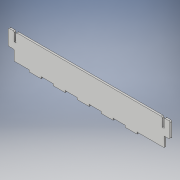
# Autodesk Inventor part: back_v2
Saved by Autodesk Inventor 2017.2 (Build 212233000, 233)
## iProperties
Created: 2017-06-09
Part Number: back_v2
Material: Generic
Document SubType Name: Modeling
Designer: SandeepSH
Density: 1 g/cm^3
Appearance: Default
Author: SandeepSH
Autodesk Inventor part; units mm, degrees
ref_plane "YZ Plane" through (0, 0, 0) normal (1, 0, 0) x (0, 1, 0)
ref_plane "XZ Plane" through (0, 0, 0) normal (0, 1, 0) x (-1, 0, 0)
ref_plane "XY Plane" through (0, 0, 0) normal (0, 0, 1) x (1, 0, 0)
sketch "Sketch1" plane through (0, 0, 0) normal (0, 0, 1) x (1, 0, 0)
  line L0 (0, 0) -> (250, 0)
  line L1 (250, 0) -> (250, 46)
  line L2 (250, 46) -> (0, 46)
  line L3 (0, 46) -> (0, 0)
  dimension "d0" = 250
  dimension "d1" = 46
  constraints: 8 end point, 2 parallel, 1 horizontal, 1 perpendicular
  measures "d0" distance of L2.end L1.end
  measures "d1" distance of L1.end L0.end
extrude "Extrusion1" add sketch "Sketch1" along normal blind 3
sketch "Sketch2" plane through (0, 0, 3) normal (0, 0, 1) x (1, 0, 0)
  line L0 (0, 0) -> (25, 0)
  line L1 (25, 0) -> (25, 3)
  line L2 (25, 3) -> (0, 3)
  line L3 (0, 3) -> (0, 0)
  line L4 (0, 0) -> (250, 0) projected
  line L5 (45, 0) -> (65, 0)
  line L6 (65, 0) -> (65, 3)
  line L7 (65, 3) -> (45, 3)
  line L8 (45, 3) -> (45, 0)
  line L9 (85, 0) -> (105, 0)
  line L10 (105, 0) -> (105, 3)
  line L11 (105, 3) -> (85, 3)
  line L12 (85, 3) -> (85, 0)
  line L13 (125, 0) -> (145, 0)
  line L14 (145, 0) -> (145, 3)
  line L15 (145, 3) -> (125, 3)
  line L16 (125, 3) -> (125, 0)
  line L17 (165, 0) -> (185, 0)
  line L18 (185, 0) -> (185, 3)
  line L19 (185, 3) -> (165, 3)
  line L20 (165, 3) -> (165, 0)
  line L21 (250, 0) -> (205, 0)
  line L22 (205, 0) -> (205, 3)
  line L23 (205, 3) -> (250, 3)
  line L24 (250, 3) -> (250, 0)
  dimension "d4" = 25
  dimension "d5" = 3
  dimension "d6" = 20
  dimension "d7" = 3
  dimension "d8" = 20
  dimension "d9" = 20
  dimension "d10" = 3
  dimension "d11" = 20
  dimension "d12" = 20
  dimension "d13" = 3
  dimension "d14" = 20
  dimension "d15" = 20
  dimension "d16" = 3
  dimension "d17" = 20
  dimension "d18" = 3
  dimension "d19" = 20
  constraints: 48 end point, 12 parallel, 6 horizontal, 6 perpendicular, 3 point on line, 1 midpoint
  measures "d4" distance of L2.end L1.end
  measures "d5" distance of L1.end L0.end
  measures "d6" distance of L7.end L6.end
  measures "d7" distance of L6.end L5.end
  measures "d8" distance between parallel lines of L8 L1
  measures "d9" distance of L11.end L10.end
  measures "d10" distance of L10.end L9.end
  measures "d11" distance from line of L11.end L6
  measures "d12" distance of L15.end L14.end
  measures "d13" distance of L14.end L13.end
  measures "d14" distance between parallel lines of L16 L10
  measures "d15" distance of L19.end L18.end
  measures "d16" distance of L18.end L17.end
  measures "d17" distance between parallel lines of L20 L14
  measures "d18" distance of L21.end L22.end
  measures "d19" distance between parallel lines of L22 L18
extrude "Extrusion2" cut sketch "Sketch2" against normal through all
sketch "Sketch3" plane through (0, 0, 3) normal (0, 0, 1) x (1, 0, 0)
  line L0 (250, 46) -> (0, 46) projected
  line L1 (0, 46) -> (3, 46)
  line L2 (3, 46) -> (3, 31)
  line L3 (3, 31) -> (0, 31)
  line L4 (0, 31) -> (0, 46)
  line L5 (250, 46) -> (247, 46)
  line L6 (247, 46) -> (247, 31)
  line L7 (247, 31) -> (250, 31)
  line L8 (250, 31) -> (250, 46)
  point P0 (0, 0)
  dimension "d22" = 3
  dimension "d23" = 15
  dimension "d24" = 3
  dimension "d25" = 15
  constraints: 16 end point, 4 parallel, 2 horizontal, 2 perpendicular
  measures "d22" distance of L2.end L3.end
  measures "d23" distance of L1.end L2.end
  measures "d24" distance of L7.end L6.end
  measures "d25" distance of L6.end L5.end
extrude "Extrusion3" cut sketch "Sketch3" against normal through all
sketch "Sketch4" plane through (0, 0, 3) normal (0, 0, 1) x (1, 0, 0)
  line L0 (247, 46) -> (3, 46) projected
  line L1 (0, 46) -> (-10, 46)
  line L2 (-10, 46) -> (-10, 20)
  line L3 (-10, 20) -> (0, 20)
  line L4 (0, 20) -> (0, 46)
  line L5 (25, 0) -> (45, 0) projected
  line L6 (250, 3) -> (250, 31) projected
  line L7 (250, 46) -> (260, 46)
  line L8 (260, 46) -> (260, 20)
  line L9 (260, 20) -> (250, 20)
  line L10 (250, 20) -> (250, 46)
  line L11 (185, 0) -> (205, 0) projected
  point P0 (0, 0)
  dimension "d28" = 10
  dimension "d29" = 20
  dimension "d30" = 10
  dimension "d31" = 20
  constraints: 16 end point, 4 parallel, 2 horizontal, 2 perpendicular
  measures "d28" distance of L3.end L2.end
  measures "d29" distance between parallel lines of L5 L3
  measures "d30" distance of L8.end L9.end
  measures "d31" distance between parallel lines of L11 L9
extrude "Extrusion4" add sketch "Sketch4" against normal blind 3
fillet "Fillet1" radius 2 10 edges at (3, 46, 1.5) (0, 46, 1.5) (-10, 46, 1.5) (-10, 20, 1.5) (0, 20, 1.5) (260, 20, 1.5) (250, 20, 1.5) (260, 46, 1.5) (247, 46, 1.5) (250, 46, 1.5) curvature continuous yes
equation "\"d11\" = d6"
equation "\"d14\" = d11"
equation "\"d17\" = d14"
equation "\"d19\" = d17"
body "Solid1"
